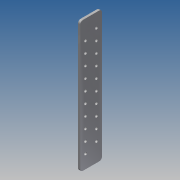
# Autodesk Inventor part: joinerBracket
Saved by Autodesk Inventor 2014 SP1 (Build 180222100, 222)
## iProperties
Created: 2014-09-15
Part Number: joinerBracket
Material: Steel
Document SubType Name: Modeling
Designer: Dave
Mass: 115.602 g
Surface Area: 125.495 cm^2
Volume: 14.7264 cm^3
Density: 7.85 g/cm^3
Appearance: Steel
Author: Dave
Autodesk Inventor part; units mm, degrees
ref_plane "YZ Plane" through (0, 0, 0) normal (1, 0, 0) x (0, 1, 0)
ref_plane "XZ Plane" through (0, 0, 0) normal (0, 1, 0) x (-1, 0, 0)
ref_plane "XY Plane" through (0, 0, 0) normal (0, 0, 1) x (1, 0, 0)
sketch "Sketch1" plane through (0, 0, 0) normal (1, 0, 0) x (0, 1, 0)
  line L0 (3.175, 0) -> (149.225, 0)
  line L1 (152.4, -3.175) -> (152.4, -22.225)
  line L2 (149.225, -25.4) -> (3.175, -25.4)
  line L3 (0, -22.225) -> (0, -3.175)
  arc A0 (152.4, -3.175) -> (149.225, 0) centre (149.225, -3.175) ccw
  arc A1 (149.225, -25.4) -> (152.4, -22.225) centre (149.225, -22.225) ccw
  arc A2 (0, -22.225) -> (3.175, -25.4) centre (3.175, -22.225) ccw
  arc A3 (3.175, 0) -> (0, -3.175) centre (3.175, -3.175) ccw
  point P0 (0, 0)
  point P1 (152.4, 0)
  point P2 (0, -25.4)
  dimension "d0" = 25.4
  dimension "d1" = 152.4
  dimension "d2" = 3.175
  constraints: 8 end point, 8 point on circle, 8 tangent, 6 point on line, 4 centre point, 3 equal radius, 2 parallel, 1 horizontal, 1 perpendicular
  measures "d0" distance of point (0, -25.4) point (0, 0)
  measures "d1" distance of point (0, 0) point (152.4, 0)
  measures "d2" radius of A0
extrude "Extrusion1" add sketch "Sketch1" along normal blind 2.54
sketch "Sketch2" plane through (2.54, 0, 0) normal (1, 0, 0) x (0, 0, -1)
  line L0 (22.225, 152.4) -> (3.175, 152.4) projected
  line L1 (0, 149.225) -> (0, 3.175) projected
  line L2 (3.175, 0) -> (22.225, 0) projected
  line L3 (25.4, 3.175) -> (25.4, 149.225) projected
  circle A0 centre (6.35, 15.5888) radius 2.5412
  line L4 (12.7, 152.4) -> (12.7, 0) construction
  circle A1 centre (19.05, 21.9388) radius 2.3772
  circle A2 centre (6.35, 28.2888) radius 2.5412
  circle A3 centre (6.35, 40.9888) radius 2.5412
  circle A4 centre (6.35, 53.6888) radius 2.5412
  circle A5 centre (6.35, 66.3888) radius 2.5412
  circle A6 centre (6.35, 79.0888) radius 2.5412
  circle A7 centre (6.35, 91.7888) radius 2.5412
  circle A8 centre (6.35, 104.4888) radius 2.5412
  circle A9 centre (6.35, 117.1888) radius 2.5412
  circle A10 centre (6.35, 129.8888) radius 2.5412
  circle A11 centre (19.05, 34.6388) radius 2.3772
  circle A12 centre (19.05, 47.3388) radius 2.3772
  circle A13 centre (19.05, 60.0388) radius 2.3772
  circle A14 centre (19.05, 72.7388) radius 2.3772
  circle A15 centre (19.05, 85.4388) radius 2.3772
  circle A16 centre (19.05, 98.1388) radius 2.3772
  circle A17 centre (19.05, 110.8388) radius 2.3772
  circle A18 centre (19.05, 123.5388) radius 2.3772
  circle A19 centre (19.05, 136.2388) radius 2.3772
  point P0 (0, 0)
  dimension "d5" = 6.35
  dimension "d6" = 12.7
  dimension "d7" = 6.35
  dimension "d10" = 12.7
  dimension "d17" = 12.7
  constraints: 20 centre point, 2 end point, 2 midpoint, 2 vertical, 36 other
  measures "d5" distance from line of A0.centre L4
  measures "d6" horizontal distance of A1.centre A0.centre
  measures "d7" vertical distance of A1.centre A0.centre
  measures "d10" distance of A0.centre A2.centre
  measures "d17" distance of A1.centre A11.centre
hole "Hole1" at (2.54, 85.4388, -19.05) at (2.54, 91.7888, -6.35) at (2.54, 98.1388, -19.05) at (2.54, 79.0888, -6.35) at (2.54, 72.7388, -19.05) at (2.54, 66.3888, -6.35) at (2.54, 60.0388, -19.05) at (2.54, 53.6888, -6.35) at (2.54, 47.3388, -19.05) at (2.54, 34.6388, -19.05) at (2.54, 21.9388, -19.05) at (2.54, 15.5888, -6.35) at (2.54, 28.2888, -6.35) at (2.54, 40.9888, -6.35) at (2.54, 110.8388, -19.05) at (2.54, 117.1888, -6.35) at (2.54, 123.5388, -19.05) at (2.54, 129.8888, -6.35) at (2.54, 136.2388, -19.05) at (2.54, 104.4888, -6.35) direction (-1, 0, 0) diameter 3.175 end through all
body "Solid1"
